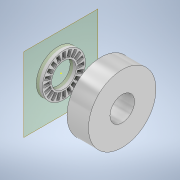
# Autodesk Inventor part: eje
Saved by Autodesk Inventor 2021 (Build 250183000, 183)
## iProperties
Created: 2021-12-11
Part Number: eje
Material: Generic
Document SubType Name: Modeling
Designer: Juan M. Casillas
Density: 1 g/cm^3
Appearance: Default
Author: Juan M. Casillas
Autodesk Inventor part; units mm, degrees
ref_plane "YZ Plane" through (0, 0, 0) normal (1, 0, 0) x (0, 1, 0)
ref_plane "XZ Plane" through (0, 0, 0) normal (0, 1, 0) x (-1, 0, 0)
ref_plane "XY Plane" through (0, 0, 0) normal (0, 0, 1) x (1, 0, 0)
sketch "Sketch1" plane through (0, 0, 0) normal (1, 0, 0) x (0, 1, 0)
  circle A0 centre (0, 0) radius 7.96
  dimension "d0" = 15.92
  constraints: 1 centre point, 1 coincident
  measures "d0" diameter of A0
extrude "Extrusion1" add sketch "Sketch1" along normal blind 8
sketch "Sketch2" plane through (8, 0, 0) normal (1, 0, 0) x (0, 0, -1)
  circle A0 centre (0, 0) radius 7.96 projected
  circle A1 centre (0, 0) radius 9.96
  dimension "d3" = 2
  constraints: 1 centre point
  measures "d3" radial gap between concentric circles of A0 A1
extrude "Extrusion2" add sketch "Sketch2" along normal blind 2
sketch "Sketch3" plane through (8, 0, 0) normal (1, 0, 0) x (0, 0, -1)
  circle A0 centre (0, 0) radius 7.96 projected
extrude "Extrusion3" add sketch "Sketch3" along normal blind 2
sketch "Sketch4" plane through (0, 0, 0) normal (-1, 0, 0) x (0, 0, 1)
  circle A0 centre (0, 0) radius 7.96 projected
  circle A1 centre (0, 0) radius 9.96
  dimension "d8" = 2
  constraints: 1 centre point
  measures "d8" radial gap between concentric circles of A0 A1
extrude "Extrusion4" add sketch "Sketch4" along normal blind 2 contours A0 | A1
sketch "Sketch5" plane through (-2, 0, 0) normal (-1, 0, 0) x (0, 0, 1)
  circle A0 centre (0, 0) radius 4
  dimension "d12" = 8
  constraints: 1 centre point
  measures "d12" diameter of A0
extrude "Extrusion5" add sketch "Sketch5" along normal blind 20
sketch "Sketch6" plane through (-22, 0, 0) normal (-1, 0, 0) x (0, 0, 1)
  circle A0 centre (0, 0) radius 4 projected
  circle A1 centre (0, 0) radius 4.5
  dimension "d15" = 0.5
  constraints: 1 centre point
  measures "d15" radial gap between concentric circles of A0 A1
extrude "Extrusion6" add sketch "Sketch6" against normal up to surface (20 mm away) separate body
sketch "Sketch7" plane through (-22, 0, 0) normal (-1, 0, 0) x (0, 0, 1)
  circle A0 centre (0, 0) radius 4 projected
extrude "Extrusion7" add sketch "Sketch7" along normal blind 40 separate body
sketch "Sketch8" plane through (-22, 0, 0) normal (-1, 0, 0) x (0, 0, 1)
  circle A0 centre (0, 0) radius 4.5 construction
  circle A1 centre (0, 0) radius 4 construction
  circle A2 centre (0, 0) radius 11
  dimension "d20" = 22
  constraints: 1 centre point, 1 coincident
  measures "d20" diameter of A2
extrude "Extrusion8" add sketch "Sketch8" along normal blind 7 separate body
sketch "Sketch9" plane through (-62, 0, 0) normal (-1, 0, 0) x (0, 0, 1)
  circle A0 centre (0, 0) radius 11
  dimension "d23" = 22
  constraints: 1 centre point, 1 coincident
  measures "d23" diameter of A0
extrude "Extrusion9" add sketch "Sketch9" against normal blind 7 separate body
sketch "Sketch10" plane through (-62, 0, 0) normal (-1, 0, 0) x (0, 0, 1)
  circle A0 centre (0, 0) radius 4.5
  dimension "d26" = 9
  constraints: 1 centre point, 1 coincident
  measures "d26" diameter of A0
extrude "Extrusion10" add sketch "Sketch10" along normal blind 2 separate body
sketch "Sketch11" plane through (-64, 0, 0) normal (-1, 0, 0) x (0, 0, 1)
  point P0 (0, 0)
  point P1 (0, 0)
  constraints: 1 coincident
hole "Hole1" at (-64, 0, 0) direction (1, 0, 0) diameter 3.42 depth 8 bodies 6
ref_plane "Work Plane1" through (-42, 0, 0) normal (-1, 0, 0) x (0, 0, 1)
sketch "Sketch15" plane through (-42, 0, 0) normal (-1, 0, 0) x (0, 0, 1)
  point P0 (0, 0)
sketch "Sketch16" plane through (-42, 0, 0) normal (-1, 0, 0) x (0, 0, 1)
  circle A0 centre (0, 0) radius 4 projected
  circle A1 centre (0, 0) radius 7
  dimension "d41" = 3
  constraints: 1 centre point
  measures "d41" radial gap between concentric circles of A0 A1
extrude "Extrusion12" add sketch "Sketch16" along normal mid plane 2 separate body
sketch "Sketch17" plane through (-43, 0, 0) normal (-1, 0, 0) x (0, 0, 1)
  circle A0 centre (0, 0) radius 4 construction
  circle A1 centre (0, 0) radius 7 construction
  line L0 (0, -4) -> (0, -7) construction
  line L1 (0.5, -6.5) -> (-0.5, -6.5)
  line L2 (-0.5, -6.5) -> (-0.5, -4.5)
  line L3 (-0.5, -4.5) -> (0.5, -4.5)
  line L4 (0.5, -4.5) -> (0.5, -6.5)
  line L5 (0.5, -6.5) -> (-0.5, -4.5) construction
  line L6 (-0.5, -6.5) -> (0.5, -4.5) construction
  line L7 (1.5331, -6.3364) -> (0.915, -4.4343)
  line L8 (0.915, -4.4343) -> (1.8661, -4.1252)
  line L9 (1.8661, -4.1252) -> (2.4841, -6.0274)
  line L10 (2.4841, -6.0274) -> (1.5331, -6.3364)
  line L11 (2.4841, -6.0274) -> (0.915, -4.4343) construction
  line L12 (1.5331, -6.3364) -> (1.8661, -4.1252) construction
  line L13 (3.4161, -5.5525) -> (2.2405, -3.9345)
  line L14 (2.2405, -3.9345) -> (3.0495, -3.3467)
  line L15 (3.0495, -3.3467) -> (4.2251, -4.9647)
  line L16 (4.2251, -4.9647) -> (3.4161, -5.5525)
  line L17 (4.2251, -4.9647) -> (2.2405, -3.9345) construction
  line L18 (3.4161, -5.5525) -> (3.0495, -3.3467) construction
  line L19 (4.9647, -4.2251) -> (3.3467, -3.0495)
  line L20 (3.3467, -3.0495) -> (3.9345, -2.2405)
  line L21 (3.9345, -2.2405) -> (5.5525, -3.4161)
  line L22 (5.5525, -3.4161) -> (4.9647, -4.2251)
  line L23 (5.5525, -3.4161) -> (3.3467, -3.0495) construction
  line L24 (4.9647, -4.2251) -> (3.9345, -2.2405) construction
  line L25 (6.0274, -2.4841) -> (4.1252, -1.8661)
  line L26 (4.1252, -1.8661) -> (4.4343, -0.915)
  line L27 (4.4343, -0.915) -> (6.3364, -1.5331)
  line L28 (6.3364, -1.5331) -> (6.0274, -2.4841)
  line L29 (6.3364, -1.5331) -> (4.1252, -1.8661) construction
  line L30 (6.0274, -2.4841) -> (4.4343, -0.915) construction
  line L31 (6.5, -0.5) -> (4.5, -0.5)
  line L32 (4.5, -0.5) -> (4.5, 0.5)
  line L33 (4.5, 0.5) -> (6.5, 0.5)
  line L34 (6.5, 0.5) -> (6.5, -0.5)
  line L35 (6.5, 0.5) -> (4.5, -0.5) construction
  line L36 (6.5, -0.5) -> (4.5, 0.5) construction
  line L37 (6.3364, 1.5331) -> (4.4343, 0.915)
  line L38 (4.4343, 0.915) -> (4.1252, 1.8661)
  line L39 (4.1252, 1.8661) -> (6.0274, 2.4841)
  line L40 (6.0274, 2.4841) -> (6.3364, 1.5331)
  line L41 (6.0274, 2.4841) -> (4.4343, 0.915) construction
  line L42 (6.3364, 1.5331) -> (4.1252, 1.8661) construction
  line L43 (5.5525, 3.4161) -> (3.9345, 2.2405)
  line L44 (3.9345, 2.2405) -> (3.3467, 3.0495)
  line L45 (3.3467, 3.0495) -> (4.9647, 4.2251)
  line L46 (4.9647, 4.2251) -> (5.5525, 3.4161)
  line L47 (4.9647, 4.2251) -> (3.9345, 2.2405) construction
  line L48 (5.5525, 3.4161) -> (3.3467, 3.0495) construction
  line L49 (4.2251, 4.9647) -> (3.0495, 3.3467)
  line L50 (3.0495, 3.3467) -> (2.2405, 3.9345)
  line L51 (2.2405, 3.9345) -> (3.4161, 5.5525)
  line L52 (3.4161, 5.5525) -> (4.2251, 4.9647)
  line L53 (3.4161, 5.5525) -> (3.0495, 3.3467) construction
  line L54 (4.2251, 4.9647) -> (2.2405, 3.9345) construction
  line L55 (2.4841, 6.0274) -> (1.8661, 4.1252)
  line L56 (1.8661, 4.1252) -> (0.915, 4.4343)
  line L57 (0.915, 4.4343) -> (1.5331, 6.3364)
  line L58 (1.5331, 6.3364) -> (2.4841, 6.0274)
  line L59 (1.5331, 6.3364) -> (1.8661, 4.1252) construction
  line L60 (2.4841, 6.0274) -> (0.915, 4.4343) construction
  line L61 (0.5, 6.5) -> (0.5, 4.5)
  line L62 (0.5, 4.5) -> (-0.5, 4.5)
  line L63 (-0.5, 4.5) -> (-0.5, 6.5)
  line L64 (-0.5, 6.5) -> (0.5, 6.5)
  line L65 (-0.5, 6.5) -> (0.5, 4.5) construction
  line L66 (0.5, 6.5) -> (-0.5, 4.5) construction
  line L67 (-1.5331, 6.3364) -> (-0.915, 4.4343)
  line L68 (-0.915, 4.4343) -> (-1.8661, 4.1252)
  line L69 (-1.8661, 4.1252) -> (-2.4841, 6.0274)
  line L70 (-2.4841, 6.0274) -> (-1.5331, 6.3364)
  line L71 (-2.4841, 6.0274) -> (-0.915, 4.4343) construction
  line L72 (-1.5331, 6.3364) -> (-1.8661, 4.1252) construction
  line L73 (-3.4161, 5.5525) -> (-2.2405, 3.9345)
  line L74 (-2.2405, 3.9345) -> (-3.0495, 3.3467)
  line L75 (-3.0495, 3.3467) -> (-4.2251, 4.9647)
  line L76 (-4.2251, 4.9647) -> (-3.4161, 5.5525)
  line L77 (-4.2251, 4.9647) -> (-2.2405, 3.9345) construction
  line L78 (-3.4161, 5.5525) -> (-3.0495, 3.3467) construction
  line L79 (-4.9647, 4.2251) -> (-3.3467, 3.0495)
  line L80 (-3.3467, 3.0495) -> (-3.9345, 2.2405)
  line L81 (-3.9345, 2.2405) -> (-5.5525, 3.4161)
  line L82 (-5.5525, 3.4161) -> (-4.9647, 4.2251)
  line L83 (-5.5525, 3.4161) -> (-3.3467, 3.0495) construction
  line L84 (-4.9647, 4.2251) -> (-3.9345, 2.2405) construction
  line L85 (-6.0274, 2.4841) -> (-4.1252, 1.8661)
  line L86 (-4.1252, 1.8661) -> (-4.4343, 0.915)
  line L87 (-4.4343, 0.915) -> (-6.3364, 1.5331)
  line L88 (-6.3364, 1.5331) -> (-6.0274, 2.4841)
  line L89 (-6.3364, 1.5331) -> (-4.1252, 1.8661) construction
  line L90 (-6.0274, 2.4841) -> (-4.4343, 0.915) construction
  line L91 (-6.5, 0.5) -> (-4.5, 0.5)
  line L92 (-4.5, 0.5) -> (-4.5, -0.5)
  line L93 (-4.5, -0.5) -> (-6.5, -0.5)
  line L94 (-6.5, -0.5) -> (-6.5, 0.5)
  line L95 (-6.5, -0.5) -> (-4.5, 0.5) construction
  line L96 (-6.5, 0.5) -> (-4.5, -0.5) construction
  line L97 (-6.3364, -1.5331) -> (-4.4343, -0.915)
  line L98 (-4.4343, -0.915) -> (-4.1252, -1.8661)
  line L99 (-4.1252, -1.8661) -> (-6.0274, -2.4841)
  line L100 (-6.0274, -2.4841) -> (-6.3364, -1.5331)
  line L101 (-6.0274, -2.4841) -> (-4.4343, -0.915) construction
  line L102 (-6.3364, -1.5331) -> (-4.1252, -1.8661) construction
  line L103 (-5.5525, -3.4161) -> (-3.9345, -2.2405)
  line L104 (-3.9345, -2.2405) -> (-3.3467, -3.0495)
  line L105 (-3.3467, -3.0495) -> (-4.9647, -4.2251)
  line L106 (-4.9647, -4.2251) -> (-5.5525, -3.4161)
  line L107 (-4.9647, -4.2251) -> (-3.9345, -2.2405) construction
  line L108 (-5.5525, -3.4161) -> (-3.3467, -3.0495) construction
  line L109 (-4.2251, -4.9647) -> (-3.0495, -3.3467)
  line L110 (-3.0495, -3.3467) -> (-2.2405, -3.9345)
  line L111 (-2.2405, -3.9345) -> (-3.4161, -5.5525)
  line L112 (-3.4161, -5.5525) -> (-4.2251, -4.9647)
  line L113 (-3.4161, -5.5525) -> (-3.0495, -3.3467) construction
  line L114 (-4.2251, -4.9647) -> (-2.2405, -3.9345) construction
  line L115 (-2.4841, -6.0274) -> (-1.8661, -4.1252)
  line L116 (-1.8661, -4.1252) -> (-0.915, -4.4343)
  line L117 (-0.915, -4.4343) -> (-1.5331, -6.3364)
  line L118 (-1.5331, -6.3364) -> (-2.4841, -6.0274)
  line L119 (-1.5331, -6.3364) -> (-1.8661, -4.1252) construction
  line L120 (-2.4841, -6.0274) -> (-0.915, -4.4343) construction
  point P0 (0, -5.5)
  point P1 (1.6996, -5.2308)
  point P2 (3.2328, -4.4496)
  point P3 (4.4496, -3.2328)
  point P4 (5.2308, -1.6996)
  point P5 (5.5, 0)
  point P6 (5.2308, 1.6996)
  point P7 (4.4496, 3.2328)
  point P8 (3.2328, 4.4496)
  point P9 (1.6996, 5.2308)
  point P10 (0, 5.5)
  point P11 (-1.6996, 5.2308)
  point P12 (-3.2328, 4.4496)
  point P13 (-4.4496, 3.2328)
  point P14 (-5.2308, 1.6996)
  point P15 (-5.5, 0)
  point P16 (-5.2308, -1.6996)
  point P17 (-4.4496, -3.2328)
  point P18 (-3.2328, -4.4496)
  point P19 (-1.6996, -5.2308)
  dimension "d44" = 1
  dimension "d45" = 2
  dimension "d48" = 360
  constraints: 242 end point, 41 midpoint, 2 parallel, 2 vertical alignment, 1 coincident, 1 horizontal, 1 perpendicular, 1 vertical, 223 other
  measures "d44" distance of L2.end L3.end
  measures "d45" distance of L1.end L2.end
extrude "Extrusion13" cut sketch "Sketch17" against normal blind 2 bodies 7
sketch "Sketch18" plane through (-29, 0, 0) normal (-1, 0, 0) x (0, 0, 1)
  circle A0 centre (0, 0) radius 4
  dimension "d52" = 8
  constraints: 1 centre point, 1 coincident
  measures "d52" diameter of A0
extrude "Extrusion14" cut sketch "Sketch18" against normal through all bodies 4
sketch "Sketch12" plane through (-42, 0, 0) normal (-1, 0, 0) x (0, 0, 1)
  circle A0 centre (0, 0) radius 7
  dimension "d37" = 14
  dimension "d40" = 8
  constraints: 1 centre point, 1 coincident
  measures "d40" diameter of A0
body "Solid7"
body "Solid8"
